Autodesk Inventor part; units mm, degrees
(part 5 of 8)
  arc A833 (80.01, 31.6865) -> (80.01, 32.7025) centre (80.01, 32.1945) ccw
  arc A834 (80.01, 32.7025) -> (80.01, 31.6865) centre (80.01, 32.1945) ccw
  line L239 (40.48, 30.852) -> (34.903, 30.852)
  arc A835 (34.903, 30.9028) -> (34.903, 30.8012) centre (34.903, 30.852) ccw
  arc A836 (40.48, 30.8012) -> (40.48, 30.9028) centre (40.48, 30.852) ccw
  line L240 (34.903, 30.852) -> (31.137, 30.852)
  arc A837 (31.137, 30.9028) -> (31.137, 30.8012) centre (31.137, 30.852) ccw
  arc A838 (34.903, 30.8012) -> (34.903, 30.9028) centre (34.903, 30.852) ccw
  line L241 (31.137, 30.852) -> (12.043, 30.852)
  arc A839 (12.043, 30.9028) -> (12.043, 30.8012) centre (12.043, 30.852) ccw
  arc A840 (31.137, 30.8012) -> (31.137, 30.9028) centre (31.137, 30.852) ccw
  line L242 (12.043, 30.852) -> (8.277, 30.852)
  arc A841 (8.277, 30.9028) -> (8.277, 30.8012) centre (8.277, 30.852) ccw
  arc A842 (12.043, 30.8012) -> (12.043, 30.9028) centre (12.043, 30.852) ccw
  line L243 (8.277, 30.852) -> (2.7, 30.852)
  arc A843 (2.7, 30.9028) -> (2.7, 30.8012) centre (2.7, 30.852) ccw
  arc A844 (8.277, 30.8012) -> (8.277, 30.9028) centre (8.277, 30.852) ccw
  line L244 (2.7, 30.852) -> (2.7, 39.252)
  arc A845 (2.7508, 39.252) -> (2.6492, 39.252) centre (2.7, 39.252) ccw
  arc A846 (2.6492, 30.852) -> (2.7508, 30.852) centre (2.7, 30.852) ccw
  line L245 (2.7, 39.252) -> (8.032, 39.252)
  arc A847 (8.032, 39.2012) -> (8.032, 39.3028) centre (8.032, 39.252) ccw
  arc A848 (2.7, 39.3028) -> (2.7, 39.2012) centre (2.7, 39.252) ccw
  line L246 (8.032, 39.252) -> (8.032, 38.952)
  arc A849 (7.9812, 38.952) -> (8.0828, 38.952) centre (8.032, 38.952) ccw
  arc A850 (8.0828, 39.252) -> (7.9812, 39.252) centre (8.032, 39.252) ccw
  line L247 (8.032, 38.952) -> (9.511, 38.952)
  arc A851 (9.511, 38.9012) -> (9.511, 39.0028) centre (9.511, 38.952) ccw
  arc A852 (8.032, 39.0028) -> (8.032, 38.9012) centre (8.032, 38.952) ccw
  line L248 (9.511, 38.952) -> (9.511, 39.252)
  arc A853 (9.5618, 39.252) -> (9.4602, 39.252) centre (9.511, 39.252) ccw
  arc A854 (9.4602, 38.952) -> (9.5618, 38.952) centre (9.511, 38.952) ccw
  line L249 (9.511, 39.252) -> (19.707, 39.252)
  arc A855 (19.707, 39.2012) -> (19.707, 39.3028) centre (19.707, 39.252) ccw
  arc A856 (9.511, 39.3028) -> (9.511, 39.2012) centre (9.511, 39.252) ccw
  line L250 (19.707, 39.252) -> (19.707, 37.702)
  arc A857 (19.6562, 37.702) -> (19.7578, 37.702) centre (19.707, 37.702) ccw
  arc A858 (19.7578, 39.252) -> (19.6562, 39.252) centre (19.707, 39.252) ccw
  line L251 (19.707, 37.702) -> (23.473, 37.702)
  arc A859 (23.473, 37.6512) -> (23.473, 37.7528) centre (23.473, 37.702) ccw
  arc A860 (19.707, 37.7528) -> (19.707, 37.6512) centre (19.707, 37.702) ccw
  line L252 (23.473, 37.702) -> (23.473, 39.252)
  arc A861 (23.5238, 39.252) -> (23.4222, 39.252) centre (23.473, 39.252) ccw
  arc A862 (23.4222, 37.702) -> (23.5238, 37.702) centre (23.473, 37.702) ccw
  line L253 (19.707, 39.252) -> (23.473, 39.252)
  arc A863 (23.473, 39.2012) -> (23.473, 39.3028) centre (23.473, 39.252) ccw
  arc A864 (19.707, 39.3028) -> (19.707, 39.2012) centre (19.707, 39.252) ccw
  line L254 (23.473, 39.252) -> (33.432, 39.252)
  arc A865 (33.432, 39.2012) -> (33.432, 39.3028) centre (33.432, 39.252) ccw
  arc A866 (23.473, 39.3028) -> (23.473, 39.2012) centre (23.473, 39.252) ccw
  line L255 (34.911, 39.252) -> (40.48, 39.252)
  arc A867 (40.48, 39.2012) -> (40.48, 39.3028) centre (40.48, 39.252) ccw
  arc A868 (34.911, 39.3028) -> (34.911, 39.2012) centre (34.911, 39.252) ccw
  line L256 (40.48, 39.252) -> (40.48, 30.852)
  arc A869 (40.4292, 30.852) -> (40.5308, 30.852) centre (40.48, 30.852) ccw
  arc A870 (40.5308, 39.252) -> (40.4292, 39.252) centre (40.48, 39.252) ccw
  line L257 (39.355, 31.777) -> (34.91, 31.777)
  arc A871 (34.91, 31.8278) -> (34.91, 31.7262) centre (34.91, 31.777) ccw
  arc A872 (39.355, 31.7262) -> (39.355, 31.8278) centre (39.355, 31.777) ccw
  line L258 (31.135, 31.777) -> (12.045, 31.777)
  arc A873 (12.045, 31.8278) -> (12.045, 31.7262) centre (12.045, 31.777) ccw
  arc A874 (31.135, 31.7262) -> (31.135, 31.8278) centre (31.135, 31.777) ccw
  line L259 (8.27, 31.777) -> (3.825, 31.777)
  arc A875 (3.825, 31.8278) -> (3.825, 31.7262) centre (3.825, 31.777) ccw
  arc A876 (8.27, 31.7262) -> (8.27, 31.8278) centre (8.27, 31.777) ccw
  line L260 (3.825, 31.777) -> (3.825, 38.327)
  arc A877 (3.8758, 38.327) -> (3.7742, 38.327) centre (3.825, 38.327) ccw
  arc A878 (3.7742, 31.777) -> (3.8758, 31.777) centre (3.825, 31.777) ccw
  line L261 (3.825, 38.327) -> (19.707, 38.327)
  arc A879 (19.707, 38.2762) -> (19.707, 38.3778) centre (19.707, 38.327) ccw
  arc A880 (3.825, 38.3778) -> (3.825, 38.2762) centre (3.825, 38.327) ccw
  line L262 (23.473, 38.327) -> (39.355, 38.327)
  arc A881 (39.355, 38.2762) -> (39.355, 38.3778) centre (39.355, 38.327) ccw
  arc A882 (23.473, 38.3778) -> (23.473, 38.2762) centre (23.473, 38.327) ccw
  line L263 (39.355, 38.327) -> (39.355, 31.777)
  arc A883 (39.3042, 31.777) -> (39.4058, 31.777) centre (39.355, 31.777) ccw
  arc A884 (39.4058, 38.327) -> (39.3042, 38.327) centre (39.355, 38.327) ccw
  line L264 (33.432, 39.252) -> (33.432, 38.952)
  arc A885 (33.3812, 38.952) -> (33.4828, 38.952) centre (33.432, 38.952) ccw
  arc A886 (33.4828, 39.252) -> (33.3812, 39.252) centre (33.432, 39.252) ccw
  line L265 (33.432, 38.952) -> (34.911, 38.952)
  arc A887 (34.911, 38.9012) -> (34.911, 39.0028) centre (34.911, 38.952) ccw
  arc A888 (33.432, 39.0028) -> (33.432, 38.9012) centre (33.432, 38.952) ccw
  line L266 (34.911, 38.952) -> (34.911, 39.252)
  arc A889 (34.9618, 39.252) -> (34.8602, 39.252) centre (34.911, 39.252) ccw
  arc A890 (34.8602, 38.952) -> (34.9618, 38.952) centre (34.911, 38.952) ccw
  line L267 (34.903, 30.852) -> (34.903, 32.402)
  arc A891 (34.9538, 32.402) -> (34.8522, 32.402) centre (34.903, 32.402) ccw
  arc A892 (34.8522, 30.852) -> (34.9538, 30.852) centre (34.903, 30.852) ccw
  line L268 (34.903, 32.402) -> (31.137, 32.402)
  arc A893 (31.137, 32.4528) -> (31.137, 32.3512) centre (31.137, 32.402) ccw
  arc A894 (34.903, 32.3512) -> (34.903, 32.4528) centre (34.903, 32.402) ccw
  line L269 (31.137, 32.402) -> (31.137, 30.852)
  arc A895 (31.0862, 30.852) -> (31.1878, 30.852) centre (31.137, 30.852) ccw
  arc A896 (31.1878, 32.402) -> (31.0862, 32.402) centre (31.137, 32.402) ccw
  line L270 (12.043, 30.852) -> (12.043, 32.402)
  arc A897 (12.0938, 32.402) -> (11.9922, 32.402) centre (12.043, 32.402) ccw
  arc A898 (11.9922, 30.852) -> (12.0938, 30.852) centre (12.043, 30.852) ccw
  line L271 (12.043, 32.402) -> (8.277, 32.402)
  arc A899 (8.277, 32.4528) -> (8.277, 32.3512) centre (8.277, 32.402) ccw
  arc A900 (12.043, 32.3512) -> (12.043, 32.4528) centre (12.043, 32.402) ccw
  line L272 (8.277, 32.402) -> (8.277, 30.852)
  arc A901 (8.2262, 30.852) -> (8.3278, 30.852) centre (8.277, 30.852) ccw
  arc A902 (8.3278, 32.402) -> (8.2262, 32.402) centre (8.277, 32.402) ccw
  line L273 (47.625, 24.13) -> (49.657, 24.13)
  arc A903 (75.8504, 60.4569) -> (77.8504, 60.4569) centre (76.8504, 60.4569) ccw
  arc A904 (75.8821, 60.4569) -> (75.8186, 60.4569) centre (75.8503, 60.4569) ccw
  arc A905 (77.8821, 60.4569) -> (77.8186, 60.4569) centre (77.8503, 60.4569) ccw
  line L274 (71.7902, 55.21) -> (72.0512, 55.4188)
  arc A906 (72.0631, 55.4039) -> (72.0393, 55.4337) centre (72.0512, 55.4188) ccw
  arc A907 (71.7783, 55.2248) -> (71.8021, 55.1951) centre (71.7902, 55.2099) ccw
  line L275 (72.0512, 55.4188) -> (72.0512, 54.479)
  arc A908 (72.0322, 54.479) -> (72.0703, 54.479) centre (72.0513, 54.479) ccw
  arc A909 (72.0703, 55.4188) -> (72.0322, 55.4188) centre (72.0513, 55.4188) ccw
  line L276 (71.7902, 54.479) -> (72.3123, 54.479)
  arc A910 (72.3123, 54.46) -> (72.3123, 54.4981) centre (72.3123, 54.4791) ccw
  arc A911 (71.7902, 54.4981) -> (71.7902, 54.46) centre (71.7902, 54.4791) ccw
  arc A912 (72.3123, 53.1839) -> (72.0773, 53.4188) centre (72.0773, 53.1838) ccw
  arc A913 (72.2932, 53.1839) -> (72.3313, 53.1839) centre (72.3123, 53.1839) ccw
  arc A914 (72.0773, 53.4379) -> (72.0773, 53.3998) centre (72.0773, 53.4189) ccw
  arc A915 (72.0773, 53.4188) -> (71.7902, 53.21) centre (72.0773, 53.117) ccw
  arc A916 (72.0773, 53.3998) -> (72.0773, 53.4379) centre (72.0773, 53.4189) ccw
  arc A917 (71.7721, 53.2158) -> (71.8083, 53.2041) centre (71.7902, 53.2099) ccw
  arc A918 (72.234, 53.0011) -> (72.3123, 53.1839) centre (72.0598, 53.1839) ccw
  arc A919 (72.2208, 53.0149) -> (72.2471, 52.9873) centre (72.2339, 53.0011) ccw
  arc A920 (72.3313, 53.1839) -> (72.2932, 53.1839) centre (72.3123, 53.1839) ccw
  line L277 (72.234, 53.0011) -> (71.7902, 52.479)
  arc A921 (71.7757, 52.4914) -> (71.8047, 52.4667) centre (71.7902, 52.4791) ccw
  arc A922 (72.2485, 52.9888) -> (72.2195, 53.0135) centre (72.234, 53.0011) ccw
  line L278 (71.7902, 52.479) -> (72.3123, 52.479)
  arc A923 (72.3123, 52.46) -> (72.3123, 52.4981) centre (72.3123, 52.4791) ccw
  arc A924 (71.7902, 52.4981) -> (71.7902, 52.46) centre (71.7902, 52.4791) ccw
  line L279 (81.2902, 52.479) -> (81.5512, 52.479)
  arc A925 (81.5512, 52.46) -> (81.5512, 52.4981) centre (81.5512, 52.4791) ccw
  arc A926 (81.2902, 52.4981) -> (81.2902, 52.46) centre (81.2902, 52.4791) ccw
  arc A927 (81.5512, 52.479) -> (81.5512, 53.0011) centre (81.5512, 52.74) ccw
  arc A928 (81.5512, 52.4981) -> (81.5512, 52.46) centre (81.5512, 52.4791) ccw
  arc A929 (81.5512, 53.0202) -> (81.5512, 52.9821) centre (81.5512, 53.0012) ccw
  line L280 (81.2902, 53.4188) -> (81.6034, 53.4188)
  arc A930 (81.6034, 53.3998) -> (81.6034, 53.4379) centre (81.6034, 53.4189) ccw
  arc A931 (81.2902, 53.4379) -> (81.2902, 53.3998) centre (81.2902, 53.4189) ccw
  arc A932 (81.6034, 53.0011) -> (81.6034, 53.4188) centre (81.6034, 53.2099) ccw
  arc A933 (81.6034, 53.0202) -> (81.6034, 52.9821) centre (81.6034, 53.0012) ccw
  arc A934 (81.6034, 53.4379) -> (81.6034, 53.3998) centre (81.6034, 53.4189) ccw
  constraints: 2077 point on circle, 935 centre point, 562 end point, 250 point on line, 27 midpoint
sketch "23" plane through (0, 0, 0) normal (0, 0, 1) x (1, 0, 0)
  point P0 (76.942, 12.1412)
  point P1 (98.4424, 74.8321)
  point P2 (98.4424, 12.1412)
  point P3 (55.2831, 53.8771)
  point P4 (33.5609, 74.9119)
  point P5 (55.3493, 12.1412)
  point P6 (12.085, 12.0469)
  point P7 (12.0477, 53.7972)
  point P8 (56.2064, 35.052)
  point P9 (12.0927, 74.8321)
  point P10 (98.4424, 53.9569)
  point P11 (76.8576, 74.8321)
  point P12 (77.4954, 35.2425)
  point P13 (21.59, 35.052)
  point P14 (15.24, 25.4)
  point P15 (33.6842, 53.9569)
  point P16 (98.4358, 32.7896)
  point P17 (33.6796, 12.0886)
  point P18 (51.181, 25.4)
  point P19 (76.8504, 53.9569)
  point P20 (55.2196, 75.0062)
sketch "25" plane through (0, 0, 0) normal (0, 0, 1) x (1, 0, 0)
  line L0 (2.6162, 64.8462) -> (2.6162, 66.4718)
  arc A0 (2.6543, 66.4718) -> (2.5781, 66.4718) centre (2.6162, 66.4718) ccw
  arc A1 (2.5781, 64.8462) -> (2.6543, 64.8462) centre (2.6162, 64.8462) ccw
  line L1 (2.6162, 66.4718) -> (3.1581, 65.5687)
  arc A2 (3.1254, 65.5491) -> (3.1907, 65.5883) centre (3.1581, 65.5687) ccw
  arc A3 (2.6489, 66.4914) -> (2.5835, 66.4522) centre (2.6162, 66.4718) ccw
  line L2 (3.1581, 65.5687) -> (3.6999, 66.4718)
  arc A4 (3.7326, 66.4522) -> (3.6673, 66.4914) centre (3.7, 66.4718) ccw
  arc A5 (3.1254, 65.5883) -> (3.1907, 65.5491) centre (3.1581, 65.5687) ccw
  line L3 (3.6999, 66.4718) -> (3.6999, 64.8462)
  arc A6 (3.6618, 64.8462) -> (3.738, 64.8462) centre (3.6999, 64.8462) ccw
  arc A7 (3.738, 66.4718) -> (3.6618, 66.4718) centre (3.6999, 66.4718) ccw
  line L4 (4.5096, 65.2978) -> (4.5096, 66.0202)
  arc A8 (4.5477, 66.0202) -> (4.4715, 66.0202) centre (4.5096, 66.0202) ccw
  arc A9 (4.4715, 65.2978) -> (4.5477, 65.2978) centre (4.5096, 65.2978) ccw
  arc A10 (5.4127, 66.0202) -> (4.5096, 66.0202) centre (4.9611, 66.0202) ccw
  arc A11 (5.3746, 66.0202) -> (5.4508, 66.0202) centre (5.4127, 66.0202) ccw
  arc A12 (4.4715, 66.0202) -> (4.5477, 66.0202) centre (4.5096, 66.0202) ccw
  line L5 (5.4127, 66.0202) -> (5.4127, 65.2978)
  arc A13 (5.3746, 65.2978) -> (5.4508, 65.2978) centre (5.4127, 65.2978) ccw
  arc A14 (5.4508, 66.0202) -> (5.3746, 66.0202) centre (5.4127, 66.0202) ccw
  arc A15 (4.5096, 65.2978) -> (5.4127, 65.2978) centre (4.9611, 65.2978) ccw
  arc A16 (4.5477, 65.2978) -> (4.4715, 65.2978) centre (4.5096, 65.2978) ccw
  arc A17 (5.4508, 65.2978) -> (5.3746, 65.2978) centre (5.4127, 65.2978) ccw
  line L6 (5.2321, 65.2074) -> (5.5933, 64.8462)
  arc A18 (5.5664, 64.8193) -> (5.6202, 64.8731) centre (5.5933, 64.8462) ccw
  arc A19 (5.259, 65.2344) -> (5.2051, 65.1805) centre (5.2321, 65.2074) ccw
  arc A20 (6.9443, 65.2978) -> (6.0412, 65.2978) centre (6.4928, 65.2978) ccw
  arc A21 (6.9062, 65.2978) -> (6.9824, 65.2978) centre (6.9443, 65.2978) ccw
  arc A22 (6.0031, 65.2978) -> (6.0793, 65.2978) centre (6.0412, 65.2978) ccw
  arc A23 (6.0412, 65.2978) -> (6.9443, 65.2978) centre (6.4928, 65.2978) ccw
  arc A24 (6.0793, 65.2978) -> (6.0031, 65.2978) centre (6.0412, 65.2978) ccw
  arc A25 (6.9824, 65.2978) -> (6.9062, 65.2978) centre (6.9443, 65.2978) ccw
  arc A26 (6.854, 66.1106) -> (6.1315, 66.1106) centre (6.4928, 66.1106) ccw
  arc A27 (6.8159, 66.1106) -> (6.8921, 66.1106) centre (6.854, 66.1106) ccw
  arc A28 (6.0934, 66.1106) -> (6.1696, 66.1106) centre (6.1315, 66.1106) ccw
  arc A29 (6.1315, 66.1106) -> (6.854, 66.1106) centre (6.4928, 66.1106) ccw
  arc A30 (6.1696, 66.1106) -> (6.0934, 66.1106) centre (6.1315, 66.1106) ccw
  arc A31 (6.8921, 66.1106) -> (6.8159, 66.1106) centre (6.854, 66.1106) ccw
  line L7 (38.1762, 64.8462) -> (38.7181, 66.4718)
  arc A32 (38.7542, 66.4598) -> (38.6819, 66.4838) centre (38.7181, 66.4718) ccw
  arc A33 (38.1401, 64.8582) -> (38.2123, 64.8342) centre (38.1762, 64.8462) ccw
  line L8 (38.7181, 66.4718) -> (39.2599, 64.8462)
  arc A34 (39.2238, 64.8342) -> (39.2961, 64.8582) centre (39.26, 64.8462) ccw
  arc A35 (38.7542, 66.4838) -> (38.6819, 66.4598) centre (38.7181, 66.4718) ccw
  line L9 (39.1245, 65.2526) -> (38.3117, 65.2526)
  arc A36 (38.3117, 65.2907) -> (38.3117, 65.2145) centre (38.3117, 65.2526) ccw
  arc A37 (39.1245, 65.2145) -> (39.1245, 65.2907) centre (39.1245, 65.2526) ccw
  line L10 (39.9686, 66.4718) -> (39.9686, 64.8462)
  arc A38 (39.9305, 64.8462) -> (40.0067, 64.8462) centre (39.9686, 64.8462) ccw
  arc A39 (40.0067, 66.4718) -> (39.9305, 66.4718) centre (39.9686, 66.4718) ccw
  line L11 (39.7879, 64.8462) -> (40.1492, 64.8462)
  arc A40 (40.1492, 64.8081) -> (40.1492, 64.8843) centre (40.1492, 64.8462) ccw
  arc A41 (39.7879, 64.8843) -> (39.7879, 64.8081) centre (39.7879, 64.8462) ccw
  line L12 (39.7879, 66.4718) -> (40.1492, 66.4718)
  arc A42 (40.1492, 66.4337) -> (40.1492, 66.5099) centre (40.1492, 66.4718) ccw
  arc A43 (39.7879, 66.5099) -> (39.7879, 66.4337) centre (39.7879, 66.4718) ccw
  line L13 (40.8288, 64.8462) -> (40.8288, 66.4718)
  arc A44 (40.8669, 66.4718) -> (40.7907, 66.4718) centre (40.8288, 66.4718) ccw
  arc A45 (40.7907, 64.8462) -> (40.8669, 64.8462) centre (40.8288, 64.8462) ccw
  line L14 (40.8288, 66.4718) -> (41.2803, 66.4718)
  arc A46 (41.2803, 66.4337) -> (41.2803, 66.5099) centre (41.2803, 66.4718) ccw
  arc A47 (40.8288, 66.5099) -> (40.8288, 66.4337) centre (40.8288, 66.4718) ccw
  arc A48 (41.2803, 65.5687) -> (41.2803, 66.4718) centre (41.2803, 66.0203) ccw
  arc A49 (41.2803, 65.6068) -> (41.2803, 65.5306) centre (41.2803, 65.5687) ccw
  arc A50 (41.2803, 66.5099) -> (41.2803, 66.4337) centre (41.2803, 66.4718) ccw
  line L15 (41.2803, 65.5687) -> (40.8288, 65.5687)
  arc A51 (40.8288, 65.6068) -> (40.8288, 65.5306) centre (40.8288, 65.5687) ccw
  arc A52 (41.2803, 65.5306) -> (41.2803, 65.6068) centre (41.2803, 65.5687) ccw
  line L16 (41.7319, 64.8462) -> (41.3706, 65.5687)
  arc A53 (41.4047, 65.5857) -> (41.3366, 65.5516) centre (41.3706, 65.5686) ccw
  arc A54 (41.6978, 64.8292) -> (41.766, 64.8632) centre (41.7319, 64.8462) ccw
  line L17 (42.3167, 64.6656) -> (43.0392, 64.6656)
  arc A55 (43.0392, 64.6275) -> (43.0392, 64.7037) centre (43.0392, 64.6656) ccw
  arc A56 (42.3167, 64.7037) -> (42.3167, 64.6275) centre (42.3167, 64.6656) ccw
  line L18 (43.7169, 65.2978) -> (43.7169, 66.0202)
  arc A57 (43.755, 66.0202) -> (43.6788, 66.0202) centre (43.7169, 66.0202) ccw
  arc A58 (43.6788, 65.2978) -> (43.755, 65.2978) centre (43.7169, 65.2978) ccw
  arc A59 (44.62, 66.0202) -> (43.7169, 66.0202) centre (44.1685, 66.0202) ccw
  arc A60 (44.5819, 66.0202) -> (44.6581, 66.0202) centre (44.62, 66.0202) ccw
  arc A61 (43.6788, 66.0202) -> (43.755, 66.0202) centre (43.7169, 66.0202) ccw
  line L19 (44.62, 66.0202) -> (44.62, 65.2978)
  arc A62 (44.5819, 65.2978) -> (44.6581, 65.2978) centre (44.62, 65.2978) ccw
  arc A63 (44.6581, 66.0202) -> (44.5819, 66.0202) centre (44.62, 66.0202) ccw
  arc A64 (43.7169, 65.2978) -> (44.62, 65.2978) centre (44.1685, 65.2978) ccw
  arc A65 (43.755, 65.2978) -> (43.6788, 65.2978) centre (43.7169, 65.2978) ccw
  arc A66 (44.6581, 65.2978) -> (44.5819, 65.2978) centre (44.62, 65.2978) ccw
  line L20 (44.4393, 65.2074) -> (44.8006, 64.8462)
  arc A67 (44.7736, 64.8193) -> (44.8275, 64.8731) centre (44.8006, 64.8462) ccw
  arc A68 (44.4663, 65.2344) -> (44.4124, 65.1805) centre (44.4393, 65.2074) ccw
  line L21 (61.0362, 64.8462) -> (61.0362, 66.4718)
  arc A69 (61.0743, 66.4718) -> (60.9981, 66.4718) centre (61.0362, 66.4718) ccw
  arc A70 (60.9981, 64.8462) -> (61.0743, 64.8462) centre (61.0362, 64.8462) ccw
  line L22 (61.0362, 66.4718) -> (61.4878, 66.4718)
  arc A71 (61.4878, 66.4337) -> (61.4878, 66.5099) centre (61.4878, 66.4718) ccw
  arc A72 (61.0362, 66.5099) -> (61.0362, 66.4337) centre (61.0362, 66.4718) ccw
  arc A73 (61.4878, 65.5687) -> (61.4878, 66.4718) centre (61.4878, 66.0203) ccw
  arc A74 (61.4878, 65.6068) -> (61.4878, 65.5306) centre (61.4878, 65.5687) ccw
  arc A75 (61.4878, 66.5099) -> (61.4878, 66.4337) centre (61.4878, 66.4718) ccw
  line L23 (61.4878, 65.5687) -> (61.0362, 65.5687)
  arc A76 (61.0362, 65.6068) -> (61.0362, 65.5306) centre (61.0362, 65.5687) ccw
  arc A77 (61.4878, 65.5306) -> (61.4878, 65.6068) centre (61.4878, 65.5687) ccw
  line L24 (62.5782, 64.8462) -> (62.5782, 66.4718)
  arc A78 (62.6163, 66.4718) -> (62.5401, 66.4718) centre (62.5782, 66.4718) ccw
  arc A79 (62.5401, 64.8462) -> (62.6163, 64.8462) centre (62.5782, 64.8462) ccw
  line L25 (62.5782, 65.7493) -> (63.4813, 65.7493)
  arc A80 (63.4813, 65.7112) -> (63.4813, 65.7874) centre (63.4813, 65.7493) ccw
  arc A81 (62.5782, 65.7874) -> (62.5782, 65.7112) centre (62.5782, 65.7493) ccw
  line L26 (63.4813, 66.4718) -> (63.4813, 64.8462)
  arc A82 (63.4432, 64.8462) -> (63.5194, 64.8462) centre (63.4813, 64.8462) ccw
  arc A83 (63.5194, 66.4718) -> (63.4432, 66.4718) centre (63.4813, 66.4718) ccw
  line L27 (105.4862, 3.8862) -> (105.4862, 5.5118)
  arc A84 (105.5243, 5.5118) -> (105.4481, 5.5118) centre (105.4862, 5.5118) ccw
  arc A85 (105.4481, 3.8862) -> (105.5243, 3.8862) centre (105.4862, 3.8862) ccw
  line L28 (105.4862, 5.5118) -> (106.0281, 4.6087)
  arc A86 (105.9954, 4.5891) -> (106.0607, 4.6283) centre (106.0281, 4.6087) ccw
  arc A87 (105.5189, 5.5314) -> (105.4535, 5.4922) centre (105.4862, 5.5118) ccw
  line L29 (106.0281, 4.6087) -> (106.5699, 5.5118)
  arc A88 (106.6026, 5.4922) -> (106.5373, 5.5314) centre (106.57, 5.5118) ccw
  arc A89 (105.9954, 4.6283) -> (106.0607, 4.5891) centre (106.0281, 4.6087) ccw
  line L30 (106.5699, 5.5118) -> (106.5699, 3.8862)
  arc A90 (106.5318, 3.8862) -> (106.608, 3.8862) centre (106.5699, 3.8862) ccw
  arc A91 (106.608, 5.5118) -> (106.5318, 5.5118) centre (106.5699, 5.5118) ccw
  line L31 (107.2959, 5.1506) -> (107.7475, 5.5118)
  arc A92 (107.7713, 5.482) -> (107.7237, 5.5416) centre (107.7475, 5.5118) ccw
  arc A93 (107.2721, 5.1803) -> (107.3197, 5.1208) centre (107.2959, 5.1506) ccw
  line L32 (107.7475, 5.5118) -> (107.7475, 3.8862)
  arc A94 (107.7094, 3.8862) -> (107.7856, 3.8862) centre (107.7475, 3.8862) ccw
  arc A95 (107.7856, 5.5118) -> (107.7094, 5.5118) centre (107.7475, 5.5118) ccw
  line L33 (107.2959, 3.8862) -> (108.1991, 3.8862)
  arc A96 (108.1991, 3.8481) -> (108.1991, 3.9243) centre (108.1991, 3.8862) ccw
  arc A97 (107.2959, 3.9243) -> (107.2959, 3.8481) centre (107.2959, 3.8862) ccw
  line L34 (105.4862, 24.2062) -> (105.4862, 25.8318)
  arc A98 (105.5243, 25.8318) -> (105.4481, 25.8318) centre (105.4862, 25.8318) ccw
  arc A99 (105.4481, 24.2062) -> (105.5243, 24.2062) centre (105.4862, 24.2062) ccw
  line L35 (105.4862, 25.8318) -> (106.0281, 24.9287)
  arc A100 (105.9954, 24.9091) -> (106.0607, 24.9483) centre (106.0281, 24.9287) ccw
  arc A101 (105.5189, 25.8514) -> (105.4535, 25.8122) centre (105.4862, 25.8318) ccw
  line L36 (106.0281, 24.9287) -> (106.5699, 25.8318)
  arc A102 (106.6026, 25.8122) -> (106.5373, 25.8514) centre (106.57, 25.8318) ccw
  arc A103 (105.9954, 24.9483) -> (106.0607, 24.9091) centre (106.0281, 24.9287) ccw
  line L37 (106.5699, 25.8318) -> (106.5699, 24.2062)
  arc A104 (106.5318, 24.2062) -> (106.608, 24.2062) centre (106.5699, 24.2062) ccw
  arc A105 (106.608, 25.8318) -> (106.5318, 25.8318) centre (106.5699, 25.8318) ccw
  arc A106 (108.1991, 25.4254) -> (107.7927, 25.8318) centre (107.7927, 25.4254) ccw
  arc A107 (108.161, 25.4254) -> (108.2372, 25.4254) centre (108.1991, 25.4254) ccw
  arc A108 (107.7927, 25.8699) -> (107.7927, 25.7937) centre (107.7927, 25.8318) ccw
  arc A109 (107.7927, 25.8318) -> (107.2959, 25.4706) centre (107.7926, 25.3097) ccw
  arc A110 (107.7927, 25.7937) -> (107.7927, 25.8699) centre (107.7927, 25.8318) ccw
  arc A111 (107.2597, 25.4823) -> (107.3322, 25.4588) centre (107.296, 25.4706) ccw
  arc A112 (108.0636, 25.1093) -> (108.1991, 25.4254) centre (107.7626, 25.4254) ccw
  arc A113 (108.0373, 25.1369) -> (108.0899, 25.0817) centre (108.0636, 25.1093) ccw
  arc A114 (108.2372, 25.4254) -> (108.161, 25.4254) centre (108.1991, 25.4254) ccw
  line L38 (108.0636, 25.1093) -> (107.2959, 24.2062)
  arc A115 (107.2669, 24.2309) -> (107.325, 24.1815) centre (107.296, 24.2062) ccw
  arc A116 (108.0926, 25.0846) -> (108.0346, 25.134) centre (108.0636, 25.1093) ccw
  line L39 (107.2959, 24.2062) -> (108.1991, 24.2062)
  arc A117 (108.1991, 24.1681) -> (108.1991, 24.2443) centre (108.1991, 24.2062) ccw
  arc A118 (107.2959, 24.2443) -> (107.2959, 24.1681) centre (107.2959, 24.2062) ccw
  line L40 (105.4862, 66.1162) -> (105.4862, 67.7418)
  arc A119 (105.5243, 67.7418) -> (105.4481, 67.7418) centre (105.4862, 67.7418) ccw
  arc A120 (105.4481, 66.1162) -> (105.5243, 66.1162) centre (105.4862, 66.1162) ccw
  line L41 (105.4862, 67.7418) -> (106.0281, 66.8387)
  arc A121 (105.9954, 66.8191) -> (106.0607, 66.8583) centre (106.0281, 66.8387) ccw
  arc A122 (105.5189, 67.7614) -> (105.4535, 67.7222) centre (105.4862, 67.7418) ccw
  line L42 (106.0281, 66.8387) -> (106.5699, 67.7418)
  arc A123 (106.6026, 67.7222) -> (106.5373, 67.7614) centre (106.57, 67.7418) ccw
  arc A124 (105.9954, 66.8583) -> (106.0607, 66.8191) centre (106.0281, 66.8387) ccw
  line L43 (106.5699, 67.7418) -> (106.5699, 66.1162)
  arc A125 (106.5318, 66.1162) -> (106.608, 66.1162) centre (106.5699, 66.1162) ccw
  arc A126 (106.608, 67.7418) -> (106.5318, 67.7418) centre (106.5699, 67.7418) ccw
  line L44 (107.2959, 66.1162) -> (107.7475, 66.1162)
  arc A127 (107.7475, 66.0781) -> (107.7475, 66.1543) centre (107.7475, 66.1162) ccw
  arc A128 (107.2959, 66.1543) -> (107.2959, 66.0781) centre (107.2959, 66.1162) ccw
  arc A129 (107.7475, 66.1162) -> (107.7475, 67.0193) centre (107.7475, 66.5678) ccw
  arc A130 (107.7475, 66.1543) -> (107.7475, 66.0781) centre (107.7475, 66.1162) ccw
  arc A131 (107.7475, 67.0574) -> (107.7475, 66.9812) centre (107.7475, 67.0193) ccw
  line L45 (107.2959, 67.7418) -> (107.8378, 67.7418)
  arc A132 (107.8378, 67.7037) -> (107.8378, 67.7799) centre (107.8378, 67.7418) ccw
  arc A133 (107.2959, 67.7799) -> (107.2959, 67.7037) centre (107.2959, 67.7418) ccw
  arc A134 (107.8378, 67.0193) -> (107.8378, 67.7418) centre (107.8378, 67.3805) ccw
  arc A135 (107.8378, 67.0574) -> (107.8378, 66.9812) centre (107.8378, 67.0193) ccw
  arc A136 (107.8378, 67.7799) -> (107.8378, 67.7037) centre (107.8378, 67.7418) ccw
  line L46 (107.8378, 67.0193) -> (107.4766, 67.0193)
  arc A137 (107.4766, 67.0574) -> (107.4766, 66.9812) centre (107.4766, 67.0193) ccw
  arc A138 (107.8378, 66.9812) -> (107.8378, 67.0574) centre (107.8378, 67.0193) ccw
  line L47 (67.3862, 64.8462) -> (67.3862, 66.4718)
  arc A139 (67.4243, 66.4718) -> (67.3481, 66.4718) centre (67.3862, 66.4718) ccw
  arc A140 (67.3481, 64.8462) -> (67.4243, 64.8462) centre (67.3862, 64.8462) ccw
  line L48 (67.3862, 66.4718) -> (67.9281, 65.5687)
  arc A141 (67.8954, 65.5491) -> (67.9607, 65.5883) centre (67.928, 65.5687) ccw
  arc A142 (67.4189, 66.4914) -> (67.3535, 66.4522) centre (67.3862, 66.4718) ccw
  line L49 (67.9281, 65.5687) -> (68.4699, 66.4718)
  arc A143 (68.5026, 66.4522) -> (68.4373, 66.4914) centre (68.4699, 66.4718) ccw
  arc A144 (67.8954, 65.5883) -> (67.9607, 65.5491) centre (67.928, 65.5687) ccw
  line L50 (68.4699, 66.4718) -> (68.4699, 64.8462)
  arc A145 (68.4318, 64.8462) -> (68.508, 64.8462) centre (68.4699, 64.8462) ccw
  arc A146 (68.508, 66.4718) -> (68.4318, 66.4718) centre (68.4699, 66.4718) ccw
  line L51 (69.5572, 66.4718) -> (69.1959, 65.2074)
  arc A147 (69.1593, 65.2179) -> (69.2326, 65.197) centre (69.196, 65.2074) ccw
  arc A148 (69.5938, 66.4613) -> (69.5206, 66.4823) centre (69.5572, 66.4718) ccw
  line L52 (69.1959, 65.2074) -> (70.0991, 65.2074)
  arc A149 (70.0991, 65.1693) -> (70.0991, 65.2455) centre (70.0991, 65.2074) ccw
  arc A150 (69.1959, 65.2455) -> (69.1959, 65.1693) centre (69.1959, 65.2074) ccw
  line L53 (69.8281, 65.5687) -> (69.8281, 64.8462)
  arc A151 (69.79, 64.8462) -> (69.8662, 64.8462) centre (69.8281, 64.8462) ccw
  arc A152 (69.8662, 65.5687) -> (69.79, 65.5687) centre (69.8281, 65.5687) ccw
  line L54 (86.4362, 45.4293) -> (86.8878, 45.4293)
  arc A153 (86.8878, 45.3912) -> (86.8878, 45.4674) centre (86.8878, 45.4293) ccw
  arc A154 (86.4362, 45.4674) -> (86.4362, 45.3912) centre (86.4362, 45.4293) ccw
  arc A155 (86.8878, 44.5262) -> (86.8878, 45.4293) centre (86.8878, 44.9778) ccw
  arc A156 (86.8878, 44.5643) -> (86.8878, 44.4881) centre (86.8878, 44.5262) ccw
  arc A157 (86.8878, 45.4674) -> (86.8878, 45.3912) centre (86.8878, 45.4293) ccw
  line L55 (86.8878, 44.5262) -> (86.4362, 44.5262)
  arc A158 (86.4362, 44.5643) -> (86.4362, 44.4881) centre (86.4362, 44.5262) ccw
  arc A159 (86.8878, 44.4881) -> (86.8878, 44.5643) centre (86.8878, 44.5262) ccw
  line L56 (86.4362, 44.5262) -> (86.4362, 46.1518)
  arc A160 (86.4743, 46.1518) -> (86.3981, 46.1518) centre (86.4362, 46.1518) ccw
  arc A161 (86.3981, 44.5262) -> (86.4743, 44.5262) centre (86.4362, 44.5262) ccw
  line L57 (86.4362, 46.1518) -> (86.8878, 46.1518)
  arc A162 (86.8878, 46.1137) -> (86.8878, 46.1899) centre (86.8878, 46.1518) ccw
  arc A163 (86.4362, 46.1899) -> (86.4362, 46.1137) centre (86.4362, 46.1518) ccw
  arc A164 (86.8878, 45.4293) -> (86.8878, 46.1518) centre (86.8878, 45.7905) ccw
  arc A165 (86.8878, 45.4674) -> (86.8878, 45.3912) centre (86.8878, 45.4293) ccw
  arc A166 (86.8878, 46.1899) -> (86.8878, 46.1137) centre (86.8878, 46.1518) ccw
  line L58 (87.8358, 44.5262) -> (88.3777, 46.1518)
  arc A167 (88.4138, 46.1398) -> (88.3415, 46.1638) centre (88.3776, 46.1518) ccw
  arc A168 (87.7997, 44.5382) -> (87.872, 44.5142) centre (87.8359, 44.5262) ccw
  line L59 (88.3777, 46.1518) -> (88.9195, 44.5262)
  arc A169 (88.8834, 44.5142) -> (88.9557, 44.5382) centre (88.9195, 44.5262) ccw
  arc A170 (88.4138, 46.1638) -> (88.3415, 46.1398) centre (88.3776, 46.1518) ccw
  line L60 (88.7841, 44.9326) -> (87.9713, 44.9326)
  arc A171 (87.9713, 44.9707) -> (87.9713, 44.8945) centre (87.9713, 44.9326) ccw
  arc A172 (88.7841, 44.8945) -> (88.7841, 44.9707) centre (88.7841, 44.9326) ccw
  line L61 (89.8366, 44.5262) -> (89.8366, 46.1518)
  arc A173 (89.8747, 46.1518) -> (89.7985, 46.1518) centre (89.8366, 46.1518) ccw
  arc A174 (89.7985, 44.5262) -> (89.8747, 44.5262) centre (89.8366, 44.5262) ccw
  line L62 (89.385, 46.1518) -> (90.2882, 46.1518)
  arc A175 (90.2882, 46.1137) -> (90.2882, 46.1899) centre (90.2882, 46.1518) ccw
  arc A176 (89.385, 46.1899) -> (89.385, 46.1137) centre (89.385, 46.1518) ccw
  line L63 (91.1913, 44.5262) -> (91.1913, 46.1518)
  arc A177 (91.2294, 46.1518) -> (91.1532, 46.1518) centre (91.1913, 46.1518) ccw
  arc A178 (91.1532, 44.5262) -> (91.2294, 44.5262) centre (91.1913, 44.5262) ccw
  line L64 (90.7398, 46.1518) -> (91.6429, 46.1518)
  arc A179 (91.6429, 46.1137) -> (91.6429, 46.1899) centre (91.6429, 46.1518) ccw
  arc A180 (90.7398, 46.1899) -> (90.7398, 46.1137) centre (90.7398, 46.1518) ccw
  arc A181 (71.7381, 41.9862) -> (72.0993, 42.3474) centre (71.7381, 42.3474) ccw
  arc A182 (71.7381, 42.0243) -> (71.7381, 41.9481) centre (71.7381, 41.9862) ccw
  arc A183 (72.1374, 42.3474) -> (72.0612, 42.3474) centre (72.0993, 42.3474) ccw
  arc A184 (71.1962, 42.212) -> (71.7381, 41.9862) centre (71.7381, 42.7494) ccw
  arc A185 (71.2233, 42.2388) -> (71.1691, 42.1851) centre (71.1962, 42.212) ccw
  arc A186 (71.7381, 41.9481) -> (71.7381, 42.0243) centre (71.7381, 41.9862) ccw
  arc A187 (71.6026, 43.6118) -> (71.2414, 43.2506) centre (71.6026, 43.2506) ccw
  arc A188 (71.6026, 43.5737) -> (71.6026, 43.6499) centre (71.6026, 43.6118) ccw
  arc A189 (71.2033, 43.2506) -> (71.2795, 43.2506) centre (71.2414, 43.2506) ccw
  arc A190 (72.009, 43.4763) -> (71.6026, 43.6118) centre (71.6026, 42.9345) ccw
  arc A191 (71.9861, 43.4459) -> (72.0319, 43.5068) centre (72.009, 43.4763) ccw
  arc A192 (71.6026, 43.6499) -> (71.6026, 43.5737) centre (71.6026, 43.6118) ccw
  arc A193 (71.2414, 43.2506) -> (71.422, 42.9345) centre (71.6082, 43.2506) ccw
  arc A194 (71.2795, 43.2506) -> (71.2033, 43.2506) centre (71.2414, 43.2506) ccw
  arc A195 (71.4026, 42.9016) -> (71.4413, 42.9673) centre (71.422, 42.9344) ccw
  arc A196 (72.0993, 42.3474) -> (71.9187, 42.6635) centre (71.7325, 42.3474) ccw
  arc A197 (72.0612, 42.3474) -> (72.1374, 42.3474) centre (72.0993, 42.3474) ccw
  arc A198 (71.938, 42.6964) -> (71.8993, 42.6307) centre (71.9186, 42.6636) ccw
  line L65 (71.9187, 42.6635) -> (71.422, 42.9345)
  arc A199 (71.4402, 42.9679) -> (71.4037, 42.901) centre (71.422, 42.9344) ccw
  arc A200 (71.9004, 42.6301) -> (71.9369, 42.697) centre (71.9186, 42.6636) ccw
  line L66 (73.0546, 41.9862) -> (73.0546, 43.6118)
  arc A201 (73.0927, 43.6118) -> (73.0165, 43.6118) centre (73.0546, 43.6118) ccw
  arc A202 (73.0165, 41.9862) -> (73.0927, 41.9862) centre (73.0546, 41.9862) ccw
  line L67 (72.603, 43.6118) -> (73.5061, 43.6118)
  arc A203 (73.5061, 43.5737) -> (73.5061, 43.6499) centre (73.5061, 43.6118) ccw
  arc A204 (72.603, 43.6499) -> (72.603, 43.5737) centre (72.603, 43.6118) ccw
  line L68 (74.8395, 41.9862) -> (74.117, 41.9862)
  arc A205 (74.117, 42.0243) -> (74.117, 41.9481) centre (74.117, 41.9862) ccw
  arc A206 (74.8395, 41.9481) -> (74.8395, 42.0243) centre (74.8395, 41.9862) ccw
  line L69 (74.117, 41.9862) -> (74.117, 43.6118)
  arc A207 (74.1551, 43.6118) -> (74.0789, 43.6118) centre (74.117, 43.6118) ccw
  arc A208 (74.0789, 41.9862) -> (74.1551, 41.9862) centre (74.117, 41.9862) ccw
  line L70 (74.117, 43.6118) -> (74.8395, 43.6118)
  arc A209 (74.8395, 43.5737) -> (74.8395, 43.6499) centre (74.8395, 43.6118) ccw
  arc A210 (74.117, 43.6499) -> (74.117, 43.5737) centre (74.117, 43.6118) ccw
  line L71 (74.117, 42.8893) -> (74.6589, 42.8893)
  arc A211 (74.6589, 42.8512) -> (74.6589, 42.9274) centre (74.6589, 42.8893) ccw
  arc A212 (74.117, 42.9274) -> (74.117, 42.8512) centre (74.117, 42.8893) ccw
  line L72 (75.4898, 41.9862) -> (75.4898, 43.6118)
  arc A213 (75.5279, 43.6118) -> (75.4517, 43.6118) centre (75.4898, 43.6118) ccw
  arc A214 (75.4517, 41.9862) -> (75.5279, 41.9862) centre (75.4898, 41.9862) ccw
  line L73 (75.4898, 43.6118) -> (75.9414, 43.6118)
  arc A215 (75.9414, 43.5737) -> (75.9414, 43.6499) centre (75.9414, 43.6118) ccw
  arc A216 (75.4898, 43.6499) -> (75.4898, 43.5737) centre (75.4898, 43.6118) ccw
  arc A217 (75.9414, 42.7087) -> (75.9414, 43.6118) centre (75.9414, 43.1603) ccw
  arc A218 (75.9414, 42.7468) -> (75.9414, 42.6706) centre (75.9414, 42.7087) ccw
  arc A219 (75.9414, 43.6499) -> (75.9414, 43.5737) centre (75.9414, 43.6118) ccw
  line L74 (75.9414, 42.7087) -> (75.4898, 42.7087)
  arc A220 (75.4898, 42.7468) -> (75.4898, 42.6706) centre (75.4898, 42.7087) ccw
  arc A221 (75.9414, 42.6706) -> (75.9414, 42.7468) centre (75.9414, 42.7087) ccw
  line L75 (77.053, 41.9862) -> (77.053, 43.6118)
  arc A222 (77.0911, 43.6118) -> (77.0149, 43.6118) centre (77.053, 43.6118) ccw
  arc A223 (77.0149, 41.9862) -> (77.0911, 41.9862) centre (77.053, 41.9862) ccw
  line L76 (77.053, 43.6118) -> (77.5045, 43.6118)
  arc A224 (77.5045, 43.5737) -> (77.5045, 43.6499) centre (77.5045, 43.6118) ccw
  arc A225 (77.053, 43.6499) -> (77.053, 43.5737) centre (77.053, 43.6118) ccw
  arc A226 (77.5045, 42.7087) -> (77.5045, 43.6118) centre (77.5045, 43.1603) ccw
  arc A227 (77.5045, 42.7468) -> (77.5045, 42.6706) centre (77.5045, 42.7087) ccw
  arc A228 (77.5045, 43.6499) -> (77.5045, 43.5737) centre (77.5045, 43.6118) ccw
  line L77 (77.5045, 42.7087) -> (77.053, 42.7087)
  arc A229 (77.053, 42.7468) -> (77.053, 42.6706) centre (77.053, 42.7087) ccw
  arc A230 (77.5045, 42.6706) -> (77.5045, 42.7468) centre (77.5045, 42.7087) ccw
  line L78 (79.3205, 41.9862) -> (78.598, 41.9862)
  arc A231 (78.598, 42.0243) -> (78.598, 41.9481) centre (78.598, 41.9862) ccw
  arc A232 (79.3205, 41.9481) -> (79.3205, 42.0243) centre (79.3205, 41.9862) ccw
  line L79 (78.598, 41.9862) -> (78.598, 43.6118)
  arc A233 (78.6361, 43.6118) -> (78.5599, 43.6118) centre (78.598, 43.6118) ccw
  arc A234 (78.5599, 41.9862) -> (78.6361, 41.9862) centre (78.598, 41.9862) ccw
  line L80 (78.598, 43.6118) -> (79.3205, 43.6118)
  arc A235 (79.3205, 43.5737) -> (79.3205, 43.6499) centre (79.3205, 43.6118) ccw
  arc A236 (78.598, 43.6499) -> (78.598, 43.5737) centre (78.598, 43.6118) ccw
  line L81 (78.598, 42.8893) -> (79.1398, 42.8893)
  arc A237 (79.1398, 42.8512) -> (79.1398, 42.9274) centre (79.1398, 42.8893) ccw
  arc A238 (78.598, 42.9274) -> (78.598, 42.8512) centre (78.598, 42.8893) ccw
  line L82 (79.9589, 41.9862) -> (79.9589, 43.6118)
  arc A239 (79.997, 43.6118) -> (79.9208, 43.6118) centre (79.9589, 43.6118) ccw
  arc A240 (79.9208, 41.9862) -> (79.997, 41.9862) centre (79.9589, 41.9862) ccw
  line L83 (79.9589, 43.6118) -> (80.4104, 43.6118)
  arc A241 (80.4104, 43.5737) -> (80.4104, 43.6499) centre (80.4104, 43.6118) ccw
  arc A242 (79.9589, 43.6499) -> (79.9589, 43.5737) centre (79.9589, 43.6118) ccw
  arc A243 (80.4104, 42.7087) -> (80.4104, 43.6118) centre (80.4104, 43.1603) ccw
  arc A244 (80.4104, 42.7468) -> (80.4104, 42.6706) centre (80.4104, 42.7087) ccw
  arc A245 (80.4104, 43.6499) -> (80.4104, 43.5737) centre (80.4104, 43.6118) ccw
  line L84 (80.4104, 42.7087) -> (79.9589, 42.7087)
  arc A246 (79.9589, 42.7468) -> (79.9589, 42.6706) centre (79.9589, 42.7087) ccw
  arc A247 (80.4104, 42.6706) -> (80.4104, 42.7468) centre (80.4104, 42.7087) ccw
  line L85 (80.862, 41.9862) -> (80.5007, 42.7087)
  arc A248 (80.5348, 42.7257) -> (80.4666, 42.6916) centre (80.5007, 42.7087) ccw
  arc A249 (80.8279, 41.9692) -> (80.896, 42.0032) centre (80.862, 41.9862) ccw
  line L86 (52.5978, 41.9862) -> (52.5978, 43.6118)
  arc A250 (52.6359, 43.6118) -> (52.5597, 43.6118) centre (52.5978, 43.6118) ccw
  arc A251 (52.5597, 41.9862) -> (52.6359, 41.9862) centre (52.5978, 41.9862) ccw
  line L87 (52.1462, 43.6118) -> (53.0493, 43.6118)
  arc A252 (53.0493, 43.5737) -> (53.0493, 43.6499) centre (53.0493, 43.6118) ccw
  arc A253 (52.1462, 43.6499) -> (52.1462, 43.5737) centre (52.1462, 43.6118) ccw
  line L88 (54.3827, 41.9862) -> (53.6602, 41.9862)
  arc A254 (53.6602, 42.0243) -> (53.6602, 41.9481) centre (53.6602, 41.9862) ccw
  arc A255 (54.3827, 41.9481) -> (54.3827, 42.0243) centre (54.3827, 41.9862) ccw
  line L89 (53.6602, 41.9862) -> (53.6602, 43.6118)
  arc A256 (53.6983, 43.6118) -> (53.6221, 43.6118) centre (53.6602, 43.6118) ccw
  arc A257 (53.6221, 41.9862) -> (53.6983, 41.9862) centre (53.6602, 41.9862) ccw
  line L90 (53.6602, 43.6118) -> (54.3827, 43.6118)
  arc A258 (54.3827, 43.5737) -> (54.3827, 43.6499) centre (54.3827, 43.6118) ccw
  arc A259 (53.6602, 43.6499) -> (53.6602, 43.5737) centre (53.6602, 43.6118) ccw
  line L91 (53.6602, 42.8893) -> (54.2021, 42.8893)
  arc A260 (54.2021, 42.8512) -> (54.2021, 42.9274) centre (54.2021, 42.8893) ccw
  arc A261 (53.6602, 42.9274) -> (53.6602, 42.8512) centre (53.6602, 42.8893) ccw
  line L92 (55.0258, 41.9862) -> (55.0258, 43.6118)
  arc A262 (55.0639, 43.6118) -> (54.9877, 43.6118) centre (55.0258, 43.6118) ccw
  arc A263 (54.9877, 41.9862) -> (55.0639, 41.9862) centre (55.0258, 41.9862) ccw
  line L93 (55.0258, 43.6118) -> (55.5677, 42.7087)
  arc A264 (55.535, 42.6891) -> (55.6004, 42.7283) centre (55.5677, 42.7087) ccw
  arc A265 (55.0585, 43.6314) -> (54.9932, 43.5922) centre (55.0259, 43.6118) ccw
  line L94 (55.5677, 42.7087) -> (56.1096, 43.6118)
  arc A266 (56.1422, 43.5922) -> (56.0769, 43.6314) centre (56.1096, 43.6118) ccw
  arc A267 (55.535, 42.7283) -> (55.6004, 42.6891) centre (55.5677, 42.7087) ccw
  line L95 (56.1096, 43.6118) -> (56.1096, 41.9862)
  arc A268 (56.0715, 41.9862) -> (56.1477, 41.9862) centre (56.1096, 41.9862) ccw
  arc A269 (56.1477, 43.6118) -> (56.0715, 43.6118) centre (56.1096, 43.6118) ccw
  line L96 (56.9088, 41.9862) -> (56.9088, 43.6118)
  arc A270 (56.9469, 43.6118) -> (56.8707, 43.6118) centre (56.9088, 43.6118) ccw
  arc A271 (56.8707, 41.9862) -> (56.9469, 41.9862) centre (56.9088, 41.9862) ccw
  line L97 (56.9088, 43.6118) -> (57.3603, 43.6118)
  arc A272 (57.3603, 43.5737) -> (57.3603, 43.6499) centre (57.3603, 43.6118) ccw
  arc A273 (56.9088, 43.6499) -> (56.9088, 43.5737) centre (56.9088, 43.6118) ccw
  arc A274 (57.3603, 42.7087) -> (57.3603, 43.6118) centre (57.3603, 43.1603) ccw
  arc A275 (57.3603, 42.7468) -> (57.3603, 42.6706) centre (57.3603, 42.7087) ccw
  arc A276 (57.3603, 43.6499) -> (57.3603, 43.5737) centre (57.3603, 43.6118) ccw
  line L98 (57.3603, 42.7087) -> (56.9088, 42.7087)
  arc A277 (56.9088, 42.7468) -> (56.9088, 42.6706) centre (56.9088, 42.7087) ccw
  arc A278 (57.3603, 42.6706) -> (57.3603, 42.7468) centre (57.3603, 42.7087) ccw
  line L99 (26.3652, 43.9928) -> (26.3652, 42.3672)
  arc A279 (26.3271, 42.3672) -> (26.4033, 42.3672) centre (26.3652, 42.3672) ccw
  arc A280 (26.4033, 43.9928) -> (26.3271, 43.9928) centre (26.3652, 43.9928) ccw
  line L100 (26.3652, 42.3672) -> (27.0877, 42.3672)
  arc A281 (27.0877, 42.3291) -> (27.0877, 42.4053) centre (27.0877, 42.3672) ccw
  arc A282 (26.3652, 42.4053) -> (26.3652, 42.3291) centre (26.3652, 42.3672) ccw
  line L101 (27.6648, 42.8188) -> (27.6648, 43.5412)
  arc A283 (27.7029, 43.5412) -> (27.6267, 43.5412) centre (27.6648, 43.5412) ccw
  arc A284 (27.6267, 42.8188) -> (27.7029, 42.8188) centre (27.6648, 42.8188) ccw
  arc A285 (28.5679, 43.5412) -> (27.6648, 43.5412) centre (28.1164, 43.5412) ccw
  arc A286 (28.5298, 43.5412) -> (28.606, 43.5412) centre (28.5679, 43.5412) ccw
  arc A287 (27.6267, 43.5412) -> (27.7029, 43.5412) centre (27.6648, 43.5412) ccw
  line L102 (28.5679, 43.5412) -> (28.5679, 42.8188)
  arc A288 (28.5298, 42.8188) -> (28.606, 42.8188) centre (28.5679, 42.8188) ccw
  arc A289 (28.606, 43.5412) -> (28.5298, 43.5412) centre (28.5679, 43.5412) ccw
  arc A290 (27.6648, 42.8188) -> (28.5679, 42.8188) centre (28.1164, 42.8188) ccw
  arc A291 (27.7029, 42.8188) -> (27.6267, 42.8188) centre (27.6648, 42.8188) ccw
  arc A292 (28.606, 42.8188) -> (28.5298, 42.8188) centre (28.5679, 42.8188) ccw
  line L103 (29.1376, 42.3672) -> (29.6795, 43.9928)
  arc A293 (29.7156, 43.9808) -> (29.6434, 44.0048) centre (29.6795, 43.9928) ccw
  arc A294 (29.1015, 42.3792) -> (29.1738, 42.3552) centre (29.1377, 42.3672) ccw
  line L104 (29.6795, 43.9928) -> (30.2214, 42.3672)
  arc A295 (30.1852, 42.3552) -> (30.2575, 42.3792) centre (30.2214, 42.3672) ccw
  arc A296 (29.7156, 44.0048) -> (29.6434, 43.9808) centre (29.6795, 43.9928) ccw
  line L105 (30.0859, 42.7736) -> (29.2731, 42.7736)
  arc A297 (29.2731, 42.8117) -> (29.2731, 42.7355) centre (29.2731, 42.7736) ccw
  arc A298 (30.0859, 42.7355) -> (30.0859, 42.8117) centre (30.0859, 42.7736) ccw
  line L106 (30.8432, 42.3672) -> (30.8432, 43.9928)
  arc A299 (30.8813, 43.9928) -> (30.8051, 43.9928) centre (30.8432, 43.9928) ccw
  arc A300 (30.8051, 42.3672) -> (30.8813, 42.3672) centre (30.8432, 42.3672) ccw
  line L107 (30.8432, 43.9928) -> (31.2947, 43.9928)
  arc A301 (31.2947, 43.9547) -> (31.2947, 44.0309) centre (31.2947, 43.9928) ccw
  arc A302 (30.8432, 44.0309) -> (30.8432, 43.9547) centre (30.8432, 43.9928) ccw
  arc A303 (31.7463, 43.5412) -> (31.2947, 43.9928) centre (31.2947, 43.5412) ccw
  arc A304 (31.7082, 43.5412) -> (31.7844, 43.5412) centre (31.7463, 43.5412) ccw
  arc A305 (31.2947, 44.0309) -> (31.2947, 43.9547) centre (31.2947, 43.9928) ccw
  line L108 (31.7463, 43.5412) -> (31.7463, 42.8188)
  arc A306 (31.7082, 42.8188) -> (31.7844, 42.8188) centre (31.7463, 42.8188) ccw
  arc A307 (31.7844, 43.5412) -> (31.7082, 43.5412) centre (31.7463, 43.5412) ccw
  arc A308 (31.2947, 42.3672) -> (31.7463, 42.8188) centre (31.2947, 42.8188) ccw
  arc A309 (31.2947, 42.4053) -> (31.2947, 42.3291) centre (31.2947, 42.3672) ccw
  arc A310 (31.7844, 42.8188) -> (31.7082, 42.8188) centre (31.7463, 42.8188) ccw
  line L109 (31.2947, 42.3672) -> (30.8432, 42.3672)
  arc A311 (30.8432, 42.4053) -> (30.8432, 42.3291) centre (30.8432, 42.3672) ccw
  arc A312 (31.2947, 42.3291) -> (31.2947, 42.4053) centre (31.2947, 42.3672) ccw
  line L110 (32.3924, 42.1866) -> (33.1149, 42.1866)
  arc A313 (33.1149, 42.1485) -> (33.1149, 42.2247) centre (33.1149, 42.1866) ccw
  arc A314 (32.3924, 42.2247) -> (32.3924, 42.1485) centre (32.3924, 42.1866) ccw
  line L111 (34.4274, 42.3672) -> (34.0662, 42.3672)
  arc A315 (34.0662, 42.4053) -> (34.0662, 42.3291) centre (34.0662, 42.3672) ccw
  arc A316 (34.4274, 42.3291) -> (34.4274, 42.4053) centre (34.4274, 42.3672) ccw
  arc A317 (33.7049, 42.7284) -> (34.0662, 42.3672) centre (34.0662, 42.7285) ccw
  arc A318 (33.743, 42.7284) -> (33.6668, 42.7284) centre (33.7049, 42.7284) ccw
  arc A319 (34.0662, 42.3291) -> (34.0662, 42.4053) centre (34.0662, 42.3672) ccw
  line L112 (33.7049, 42.7284) -> (33.7049, 43.6316)
  arc A320 (33.743, 43.6316) -> (33.6668, 43.6316) centre (33.7049, 43.6316) ccw
  arc A321 (33.6668, 42.7284) -> (33.743, 42.7284) centre (33.7049, 42.7284) ccw
  arc A322 (34.0662, 43.9928) -> (33.7049, 43.6316) centre (34.0662, 43.6315) ccw
  arc A323 (34.0662, 43.9547) -> (34.0662, 44.0309) centre (34.0662, 43.9928) ccw
  arc A324 (33.6668, 43.6316) -> (33.743, 43.6316) centre (33.7049, 43.6316) ccw
  line L113 (34.0662, 43.9928) -> (34.4274, 43.9928)
  arc A325 (34.4274, 43.9547) -> (34.4274, 44.0309) centre (34.4274, 43.9928) ccw
  arc A326 (34.0662, 44.0309) -> (34.0662, 43.9547) centre (34.0662, 43.9928) ccw
  line L114 (35.7891, 42.3672) -> (35.0666, 42.3672)
  arc A327 (35.0666, 42.4053) -> (35.0666, 42.3291) centre (35.0666, 42.3672) ccw
  arc A328 (35.7891, 42.3291) -> (35.7891, 42.4053) centre (35.7891, 42.3672) ccw
  line L115 (35.0666, 42.3672) -> (35.0666, 43.9928)
  arc A329 (35.1047, 43.9928) -> (35.0285, 43.9928) centre (35.0666, 43.9928) ccw
  arc A330 (35.0285, 42.3672) -> (35.1047, 42.3672) centre (35.0666, 42.3672) ccw
  line L116 (35.0666, 43.9928) -> (35.7891, 43.9928)
  arc A331 (35.7891, 43.9547) -> (35.7891, 44.0309) centre (35.7891, 43.9928) ccw
  arc A332 (35.0666, 44.0309) -> (35.0666, 43.9547) centre (35.0666, 43.9928) ccw
  line L117 (35.0666, 43.2703) -> (35.6084, 43.2703)
  arc A333 (35.6084, 43.2322) -> (35.6084, 43.3084) centre (35.6084, 43.2703) ccw
  arc A334 (35.0666, 43.3084) -> (35.0666, 43.2322) centre (35.0666, 43.2703) ccw
  line L118 (36.4213, 43.9928) -> (36.4213, 42.3672)
  arc A335 (36.3832, 42.3672) -> (36.4594, 42.3672) centre (36.4213, 42.3672) ccw
  arc A336 (36.4594, 43.9928) -> (36.3832, 43.9928) centre (36.4213, 43.9928) ccw
  line L119 (36.4213, 42.3672) -> (37.1438, 42.3672)
  arc A337 (37.1438, 42.3291) -> (37.1438, 42.4053) centre (37.1438, 42.3672) ccw
  arc A338 (36.4213, 42.4053) -> (36.4213, 42.3291) centre (36.4213, 42.3672) ccw
  line L120 (37.776, 43.9928) -> (37.776, 42.3672)
  arc A339 (37.7379, 42.3672) -> (37.8141, 42.3672) centre (37.776, 42.3672) ccw
  arc A340 (37.8141, 43.9928) -> (37.7379, 43.9928) centre (37.776, 43.9928) ccw
  line L121 (37.776, 42.3672) -> (38.4985, 42.3672)
  arc A341 (38.4985, 42.3291) -> (38.4985, 42.4053) centre (38.4985, 42.3672) ccw
  arc A342 (37.776, 42.4053) -> (37.776, 42.3291) centre (37.776, 42.3672) ccw
  arc A343 (39.5654, 42.3672) -> (39.9266, 42.7284) centre (39.5654, 42.7284) ccw
  arc A344 (39.5654, 42.4053) -> (39.5654, 42.3291) centre (39.5654, 42.3672) ccw
  arc A345 (39.9647, 42.7284) -> (39.8885, 42.7284) centre (39.9266, 42.7284) ccw
  arc A346 (39.0235, 42.593) -> (39.5654, 42.3672) centre (39.5654, 43.1304) ccw
  arc A347 (39.0506, 42.6198) -> (38.9965, 42.5661) centre (39.0235, 42.5929) ccw
  arc A348 (39.5654, 42.3291) -> (39.5654, 42.4053) centre (39.5654, 42.3672) ccw
  arc A349 (39.4299, 43.9928) -> (39.0687, 43.6316) centre (39.4299, 43.6316) ccw
  arc A350 (39.4299, 43.9547) -> (39.4299, 44.0309) centre (39.4299, 43.9928) ccw
  arc A351 (39.0306, 43.6316) -> (39.1068, 43.6316) centre (39.0687, 43.6316) ccw
  arc A352 (39.8363, 43.8573) -> (39.4299, 43.9928) centre (39.4299, 43.3155) ccw
  arc A353 (39.8135, 43.8269) -> (39.8592, 43.8878) centre (39.8363, 43.8573) ccw
  arc A354 (39.4299, 44.0309) -> (39.4299, 43.9547) centre (39.4299, 43.9928) ccw
  arc A355 (39.0687, 43.6316) -> (39.2493, 43.3155) centre (39.4355, 43.6316) ccw
  arc A356 (39.1068, 43.6316) -> (39.0306, 43.6316) centre (39.0687, 43.6316) ccw
  arc A357 (39.2299, 43.2826) -> (39.2686, 43.3483) centre (39.2493, 43.3154) ccw
  arc A358 (39.9266, 42.7284) -> (39.746, 43.0445) centre (39.5598, 42.7284) ccw
  arc A359 (39.8885, 42.7284) -> (39.9647, 42.7284) centre (39.9266, 42.7284) ccw
  arc A360 (39.7653, 43.0774) -> (39.7267, 43.0117) centre (39.746, 43.0446) ccw
  line L122 (39.746, 43.0445) -> (39.2493, 43.3155)
  arc A361 (39.2675, 43.3489) -> (39.231, 43.282) centre (39.2493, 43.3154) ccw
  arc A362 (39.7278, 43.0111) -> (39.7642, 43.078) centre (39.746, 43.0446) ccw
  line L123 (9.6012, 41.9862) -> (9.6012, 43.6118)
  arc A363 (9.6393, 43.6118) -> (9.5631, 43.6118) centre (9.6012, 43.6118) ccw
  arc A364 (9.5631, 41.9862) -> (9.6393, 41.9862) centre (9.6012, 41.9862) ccw
  line L124 (9.6012, 43.6118) -> (10.1431, 42.7087)
  arc A365 (10.1104, 42.6891) -> (10.1757, 42.7283) centre (10.1431, 42.7087) ccw
  arc A366 (9.6339, 43.6314) -> (9.5685, 43.5922) centre (9.6012, 43.6118) ccw
  line L125 (10.1431, 42.7087) -> (10.6849, 43.6118)
  arc A367 (10.7176, 43.5922) -> (10.6523, 43.6314) centre (10.685, 43.6118) ccw
  arc A368 (10.1104, 42.7283) -> (10.1757, 42.6891) centre (10.1431, 42.7087) ccw
  line L126 (10.6849, 43.6118) -> (10.6849, 41.9862)
  arc A369 (10.6468, 41.9862) -> (10.723, 41.9862) centre (10.6849, 41.9862) ccw
  arc A370 (10.723, 43.6118) -> (10.6468, 43.6118) centre (10.6849, 43.6118) ccw
  line L127 (11.4946, 42.4378) -> (11.4946, 43.1602)
  arc A371 (11.5327, 43.1602) -> (11.4565, 43.1602) centre (11.4946, 43.1602) ccw
  arc A372 (11.4565, 42.4378) -> (11.5327, 42.4378) centre (11.4946, 42.4378) ccw
  arc A373 (12.3977, 43.1602) -> (11.4946, 43.1602) centre (11.9461, 43.1602) ccw
  arc A374 (12.3596, 43.1602) -> (12.4358, 43.1602) centre (12.3977, 43.1602) ccw
  arc A375 (11.4565, 43.1602) -> (11.5327, 43.1602) centre (11.4946, 43.1602) ccw
  line L128 (12.3977, 43.1602) -> (12.3977, 42.4378)
  arc A376 (12.3596, 42.4378) -> (12.4358, 42.4378) centre (12.3977, 42.4378) ccw
  arc A377 (12.4358, 43.1602) -> (12.3596, 43.1602) centre (12.3977, 43.1602) ccw
  arc A378 (11.4946, 42.4378) -> (12.3977, 42.4378) centre (11.9461, 42.4378) ccw
  arc A379 (11.5327, 42.4378) -> (11.4565, 42.4378) centre (11.4946, 42.4378) ccw
  arc A380 (12.4358, 42.4378) -> (12.3596, 42.4378) centre (12.3977, 42.4378) ccw
  line L129 (12.2171, 42.3474) -> (12.5783, 41.9862)
  arc A381 (12.5514, 41.9593) -> (12.6052, 42.0131) centre (12.5783, 41.9862) ccw
  arc A382 (12.244, 42.3744) -> (12.1901, 42.3205) centre (12.2171, 42.3475) ccw
  line L130 (13.0262, 43.4312) -> (13.0262, 43.6118)
  arc A383 (13.0643, 43.6118) -> (12.9881, 43.6118) centre (13.0262, 43.6118) ccw
  arc A384 (12.9881, 43.4312) -> (13.0643, 43.4312) centre (13.0262, 43.4312) ccw
  line L131 (13.0262, 43.6118) -> (13.9293, 43.6118)
  arc A385 (13.9293, 43.5737) -> (13.9293, 43.6499) centre (13.9293, 43.6118) ccw
  arc A386 (13.0262, 43.6499) -> (13.0262, 43.5737) centre (13.0262, 43.6118) ccw
  arc A387 (13.441, 41.9964) -> (13.5144, 41.976) centre (13.4777, 41.9862) ccw
  arc A388 (13.966, 43.6016) -> (13.8926, 43.622) centre (13.9293, 43.6118) ccw
  line L132 (18.8722, 3.1242) -> (18.8722, 4.7498)
  arc A389 (18.9103, 4.7498) -> (18.8341, 4.7498) centre (18.8722, 4.7498) ccw
  arc A390 (18.8341, 3.1242) -> (18.9103, 3.1242) centre (18.8722, 3.1242) ccw
  line L133 (18.8722, 4.7498) -> (19.4141, 3.8467)
  arc A391 (19.3814, 3.8271) -> (19.4467, 3.8663) centre (19.414, 3.8467) ccw
  arc A392 (18.9049, 4.7694) -> (18.8395, 4.7302) centre (18.8722, 4.7498) ccw
  line L134 (19.4141, 3.8467) -> (19.9559, 4.7498)